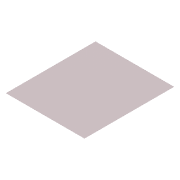
# Autodesk Inventor part: plinth
Saved by Autodesk Inventor 2017 (Build 210142000, 142)
## iProperties
Created: 2014-03-11
Part Number: plinth
Material: Glass
Document SubType Name: Modeling
Designer: Dave
Density: 2.18 g/cm^3
Appearance: Clear
Mass: 9837.25 g
Surface Area: 18240 cm^2
Volume: 4512.5 cm^3
Author: Dave
Autodesk Inventor part; units mm, degrees
ref_plane "YZ Plane" through (0, 0, 0) normal (1, 0, 0) x (0, 1, 0)
ref_plane "XZ Plane" through (0, 0, 0) normal (0, 1, 0) x (-1, 0, 0)
ref_plane "XY Plane" through (0, 0, 0) normal (0, 0, 1) x (1, 0, 0)
sketch "Sketch1" plane through (0, 0, 0) normal (0, 1, 0) x (-1, 0, 0)
  line L0 (-361.95, -412.75) -> (361.95, -412.75)
  line L1 (361.95, -412.75) -> (361.95, 412.75)
  line L2 (361.95, 412.75) -> (-361.95, 412.75)
  line L3 (-361.95, 412.75) -> (-361.95, -412.75)
  line L4 (0, 0) -> (-1302.0904, 0) construction
  line L5 (0, 0) -> (0, -698.5) construction
  dimension "d0" = 723.9
  dimension "d1" = 825.5
  constraints: 12 end point, 2 parallel, 1 coincident, 1 horizontal, 1 perpendicular, 1 vertical, 2 other
  measures "d0" distance of L2.end L1.end
  measures "d1" distance of L2.end L0.start
extrude "Extrusion1" add sketch "Sketch1" along normal blind 0.5
body "Solid1"
